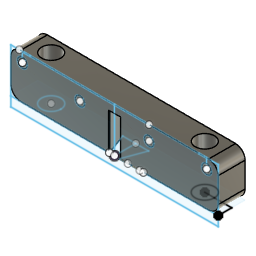
tool_holder_double_syringe v8 (Autodesk Fusion 360 design; units mm, degrees)
Autodesk Fusion 360 part; units mm, degrees
note: some values were not read from the file. Set by a fixed rule: which sketch regions a step uses.
sketch "Sketch1" plane through (0, 0, 0) normal (0, 1, 0) x (1, 0, 0)
  line L0 (0, -23) -> (44, -23)
  line L1 (44, -23) -> (46.8, -23)
  line L2 (44, -23) -> (54, -23)
  line L3 (46.8, -23) -> (48, -23)
  circle A0 centre (48, -18) radius 2.485
  line L4 (54, -23) -> (54, 0)
  line L5 (54, 0) -> (0, 0)
  line L6 (0, -23) -> (-44, -23)
  line L7 (-44, -23) -> (-46.8, -23)
  line L8 (-46.8, -23) -> (-49.55, -23)
  line L9 (-44, -23) -> (-54, -23)
  line L10 (-54, -23) -> (-54, 0)
  circle A1 centre (-48, -18) radius 2.485
  line L11 (-54, 0) -> (0, 0)
  line L12 (0, -23) -> (18, -23)
  circle A2 centre (18, -15.6) radius 2.425
  line L13 (0, -23) -> (0, 0)
  circle A3 centre (-18, -15.6) radius 2.425
  line L14 (54, 0) -> (54, 5)
  line L15 (-54, 0) -> (-54, 5)
  line L16 (-54, 5) -> (54, 5)
  line L17 (48, -23) -> (48, -18)
  line L18 (0, -23) -> (-44, -23)
  line L19 (-44, -23) -> (-48, -23)
  line L20 (-48, -23) -> (-48, -18)
  dimension "d1" = 44
  dimension "d6" = 2.8
  dimension "d8" = 10
  dimension "d10" = 1.2
  dimension "d11" = 4.97
  dimension "d14" = 23
  dimension "d38" = 4.97
  dimension "d53" = 18
  dimension "d54" = 7.4
  dimension "d55" = 4.85
  dimension "d58" = 44
  dimension "d59" = 4
  constraint horizontal L0
  constraint perpendicular L2 L4
  constraint coincident L5.end L11.end
  constraint perpendicular L4 L5
  constraint parallel L0 L12
  constraint perpendicular L11 L13
  constraint symmetric A2 L13 A3
  constraint perpendicular L5 L14
  constraint perpendicular L11 L15
  constraint perpendicular L14 L16
  constraint perpendicular L3 L17
  constraint parallel L7 L18
  constraint parallel L8 L19
  constraint perpendicular L9 L20
  measures "d1" distance of L0.start L0.end
  measures "d6" distance of L0.end L1.end
  measures "d8" distance of L0.end L2.end
  measures "d10" distance of L1.end L3.end
  measures "d11" diameter of A0
  measures "d14" distance of L2.end L4.end
  measures "d38" diameter of A1
  measures "d53" distance of L0.start L12.end
  measures "d54" distance of L12.end A2.centre
  measures "d55" diameter of A2
  measures "d58" distance of L0.start L6.end
  measures "d59" distance of L6.end L19.end
extrude "Extrude1" add sketch "Sketch1" along normal blind 14 contours L0 L1 L2 L3 L4 L5 L12 L13 | L6 L7 L8 L9 L10 L11 L13 L18 L19 | A2 | A3
sketch "bottom" plane through (0, 0, 0) normal (0, 0, -1) x (1, 0, 0)
  line L0 (54, 0) -> (-54, 0)
  line L1 (-54, 0) -> (-54, -14)
  line L2 (-54, -14) -> (54, -14)
  line L3 (54, -14) -> (54, 0)
  line L4 (0, 0) -> (7, 0)
  line L5 (0, 0) -> (2.725, 0)
  line L6 (2.725, 0) -> (15.038, 0) construction
  line L7 (0, 0) -> (-2.725, 0)
  line L8 (54, 0) -> (54, -7)
  line L9 (54, -7) -> (40, -7)
  circle A0 centre (40, -7) radius 5
  circle A1 centre (-40, -7) radius 5
  line L10 (2.725, 0) -> (14.963, 0) construction
  line L11 (0, 0) -> (-2.725, 0)
  line L12 (0, 0) -> (0, -11)
  line L13 (2.725, 0) -> (6.7287, -11)
  line L14 (2.725, 0) -> (13.1687, 0) construction
  line L15 (0, -11) -> (6.7287, -11)
  line L16 (-2.725, 0) -> (-6.7287, -11)
  line L17 (0, 0) -> (-2.725, 0)
  line L18 (0, -11) -> (-6.7287, -11)
  dimension "d17" = 2.725
  dimension "d30" = 7
  dimension "d31" = 14
  dimension "d32" = 10
  dimension "d47" = 11
  dimension "d48" = 70
  constraint coincident L4.start L5.start
  constraint parallel L0 L4
  constraint horizontal L6
  constraint coincident L0.start L3.end
  constraint perpendicular L0 L8
  constraint perpendicular L3 L9
  constraint coincident L9.end A0.centre
  constraint horizontal L10
  constraint perpendicular L4 L12
  constraint horizontal L14
  constraint perpendicular L12 L15
  constraint symmetric L4.start L12 L5.start
  constraint symmetric L5.end L12 L7.end
  constraint symmetric L15.start L12 L18.start
  constraint symmetric L12 L13.end L16.end
  measures "d17" distance of L4.start L5.end
  measures "d30" distance of L0.start L8.end
  measures "d31" distance of L8.end L9.end
  measures "d32" diameter of A0
  measures "d47" distance of L4.start L12.end
  measures "d48" angle of L13 L14
extrude "Extrude3" cut sketch "bottom" against normal blind 23 contours A0 | A1
fillet "Fillet5" radius 5 4 edges at (-54, 7, 23) (54, 7, 23) (-54, 7, 0) (54, 7, 0)
extrude "Extrude4" cut sketch "bottom" against normal blind 19 contours L0 L4 L5 L12 L13 L15 | L0 L7 L11 L12 L16 L17 L18
fillet "Fillet8" radius 1 2 edges at (-6.7287, 11, 9.5) (6.7287, 11, 9.5)
fillet "Fillet9" radius 0.3 2 edges at (-2.725, 0, 9.5) (2.725, 0, 9.5)
extrude "Extrude5" cut sketch "Sketch1" along normal blind 4 contours A2 | A3
